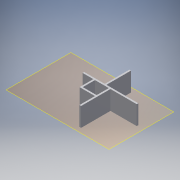
# Autodesk Inventor part: Wände_oben
Saved by Autodesk Inventor 2017 (Build 210142000, 142)
## iProperties
Created: 2017-06-01
Part Number: Wände_oben
Material: Beton
Document SubType Name: Modeling
Designer: Fake
Density: 2.40731 g/cm^3
Appearance: Weiß
Author: Fake
Autodesk Inventor part; units mm, degrees
ref_plane "YZ Plane" through (0, 0, 0) normal (1, 0, 0) x (0, 1, 0)
ref_plane "XZ Plane" through (0, 0, 0) normal (0, 1, 0) x (-1, 0, 0)
ref_plane "XY Plane" through (0, 0, 0) normal (0, 0, 1) x (1, 0, 0)
ref_plane "Arbeitsebene1" through (0, 0, 0) normal (0, 0, 1) x (1, 0, 0)
sketch "Skizze1" plane through (0, 0, 0) normal (0, 0, 1) x (1, 0, 0)
  line L0 (5680, -3575) -> (5680, 3575) projected
  line L1 (5680, 3575) -> (-5680, 3575) projected
  line L2 (-5680, 3575) -> (-5680, -3575) projected
  line L3 (-5680, -3575) -> (5680, -3575) projected
  line L4 (1400, 3375) -> (1600, 3375)
  line L5 (1600, 3375) -> (1600, 395)
  line L6 (1400, 395) -> (1400, 3375)
  line L7 (-1100, 395) -> (-1100, 195)
  line L8 (5480, 195) -> (5480, 395)
  line L9 (2290, 195) -> (2290, -3375)
  line L10 (2290, -3375) -> (2090, -3375)
  line L11 (5480, 395) -> (1600, 395)
  line L12 (1400, 395) -> (-1100, 395)
  line L13 (2290, 195) -> (5480, 195)
  line L14 (2090, -1282.3157) -> (410, -1282.3157)
  line L15 (210, -646.2385) -> (210, -1482.3157)
  line L16 (210, -1482.3157) -> (2090, -1482.3157)
  line L17 (210, 195) -> (210, -646.2385)
  line L18 (410, -1282.3157) -> (410, 195)
  line L19 (2090, -3375) -> (2090, -1482.3157)
  line L20 (2090, -1282.3157) -> (2090, 195)
  line L21 (-1100, 195) -> (210, 195)
  line L22 (410, 195) -> (2090, 195)
  dimension "d1" = 200
  dimension "d2" = 200
  dimension "d3" = 200
  dimension "d4" = 2980
  dimension "d6" = 200
  dimension "d8" = 200
  dimension "d9" = 2500
  dimension "d16" = 3880
  dimension "d26" = 200
  dimension "d27" = 200
  dimension "d28" = 1310
  dimension "d29" = 200
  dimension "d31" = 1680
  constraints: 38 end point, 12 parallel, 4 collinear, 4 horizontal, 4 perpendicular
  measures "d1" distance between parallel lines of L11 L13
  measures "d2" distance between parallel lines of L0 L8
  measures "d3" distance between parallel lines of L1 L4
  measures "d4" distance between parallel lines of L11 L4
  measures "d6" distance between parallel lines of L3 L10
  measures "d8" distance between parallel lines of L5 L6
  measures "d9" distance of L6.start L7.start
  measures "d16" distance between parallel lines of L5 L8
  measures "d26" distance between parallel lines of L18 L17
  measures "d27" distance between parallel lines of L16 L14
  measures "d28" distance between parallel lines of L17 L7
  measures "d29" distance between parallel lines of L19 L9
  measures "d31" distance between parallel lines of L20 L18
extrude "Extrusion4" add sketch "Skizze1" along normal blind 2300 contours L4 L5 L11 L8 L13 L9 L10 L19 L16 L15 L17 L21 L7 L12 L6
sketch "Skizze4" plane through (1400, 395, 0) normal (-1, 0, 0) x (0, 0, 1)
  line L0 (0, 0) -> (0, 2980) projected
  line L1 (0, 0) -> (2300, 0) projected
  line L2 (2300, 2980) -> (2300, 0) projected
  line L3 (0, 2980) -> (2300, 2980) projected
  line L4 (0, 0) -> (0, 2980) projected
  line L5 (0, 1862.9475) -> (1900, 1862.9475)
  line L6 (1900, 1862.9475) -> (1900, 912.9475)
  line L7 (1900, 912.9475) -> (0, 912.9475)
  line L8 (0, 912.9475) -> (0, 1862.9475)
  dimension "d34" = 950
  dimension "d35" = 1900
  constraints: 8 end point, 2 parallel, 1 horizontal, 1 perpendicular, 1 point on line
  measures "d34" distance of L5.end L6.end
  measures "d35" distance of L5.start L5.end
extrude "Extrusion5" cut sketch "Skizze4" against normal up to surface (200 mm away) contours L0 L5 L6 L7
sketch "Skizze5" plane through (-1100, 395, 0) normal (0, 1, 0) x (1, 0, 0)
  line L0 (0, 0) -> (2500, 0) projected
  line L1 (0, 0) -> (0, -2300) projected
  line L2 (2500, -2300) -> (0, -2300) projected
  line L3 (2500, 0) -> (2500, -2300) projected
  line L4 (0, 0) -> (2500, 0) projected
  line L5 (2437.1725, 0) -> (1487.1725, 0)
  line L6 (1487.1725, 0) -> (1487.1725, -1900)
  line L7 (1487.1725, -1900) -> (2437.1725, -1900)
  line L8 (2437.1725, -1900) -> (2437.1725, 0)
  dimension "d38" = 950
  dimension "d39" = 1900
  constraints: 8 end point, 2 parallel, 1 horizontal, 1 perpendicular, 1 point on line
  measures "d38" distance of L6.end L7.end
  measures "d39" distance of L7.end L5.start
extrude "Extrusion6" cut sketch "Skizze5" against normal up to surface (200 mm away) contours L0 L8 L7 L6
sketch "Skizze6" plane through (2090, -1282.3157, 0) normal (-1, 0, 0) x (0, 0, 1)
  line L0 (0, 0) -> (0, 1477.3157) projected
  line L1 (0, 0) -> (2300, 0) projected
  line L2 (2300, 1477.3157) -> (2300, 0) projected
  line L3 (0, 1477.3157) -> (2300, 1477.3157) projected
  line L4 (0, 0) -> (0, 1477.3157) projected
  line L5 (0, 1226.2205) -> (1900, 1226.2205)
  line L6 (1900, 1226.2205) -> (1900, 276.2205)
  line L7 (1900, 276.2205) -> (0, 276.2205)
  line L8 (0, 276.2205) -> (0, 1226.2205)
  dimension "d42" = 950
  dimension "d43" = 1900
  constraints: 8 end point, 2 parallel, 1 horizontal, 1 perpendicular, 1 point on line
  measures "d42" distance of L5.end L6.end
  measures "d43" distance of L6.end L7.end
extrude "Extrusion7" cut sketch "Skizze6" against normal up to surface (200 mm away) contours L0 L5 L6 L7
sketch "Skizze7" plane through (410, -1282.3157, 0) normal (0, 1, 0) x (1, 0, 0)
  line L0 (0, 0) -> (1680, 0) projected
  line L1 (0, 0) -> (0, -2300) projected
  line L2 (1680, -2300) -> (0, -2300) projected
  line L3 (1680, 0) -> (1680, -2300) projected
  line L4 (0, 0) -> (1680, 0) projected
  line L5 (1524.3394, 0) -> (574.3394, 0)
  line L6 (574.3394, 0) -> (574.3394, -1900)
  line L7 (574.3394, -1900) -> (1524.3394, -1900)
  line L8 (1524.3394, -1900) -> (1524.3394, 0)
  dimension "d46" = 950
  dimension "d47" = 1900
  constraints: 8 end point, 2 parallel, 1 horizontal, 1 perpendicular, 1 point on line
  measures "d46" distance of L6.end L7.end
  measures "d47" distance of L5.end L6.end
extrude "Extrusion8" cut sketch "Skizze7" against normal up to surface (200 mm away) contours L0 L8 L7 L6
